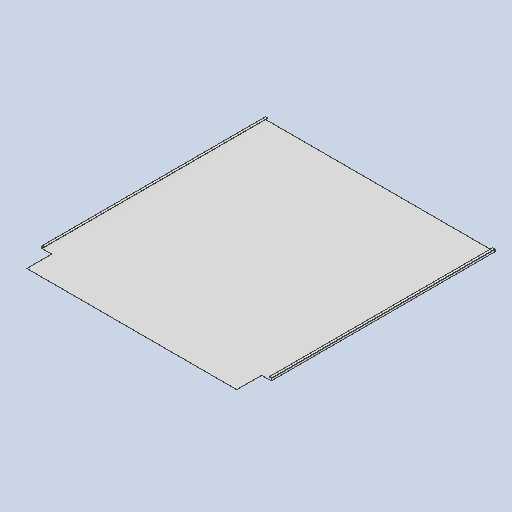
# Autodesk Inventor part: MSC 0201 sheet gills
Saved by Autodesk Inventor 2025 (Build 290162010, 162A)
## iProperties
Created: 2024-06-15
Part Number: MSC 0201 sheet gills
Material: Stainless Steel
Document SubType Name: Sheet Metal
Designer: pokla
Stock Number: МОО 0101 лист жабра
Mass: 7357.89 g
Surface Area: 36818.7 cm^2
Volume: 919.736 cm^3
Density: 8 g/cm^3
Flat Pattern Width: 96.1524 cm
Flat Pattern Length: 100 cm
Flat Pattern Area: 9615.24 cm^2
Sheet Metal Rule: Default_mm
Sheet Metal Width: 961,524 mm
Sheet Metal Length: 1000,000 mm
Sheet Metal Area: 961523,893 mm^2
Appearance: Default
Author: pokla
Autodesk Inventor part; units mm, degrees
ref_plane "YZ Plane" through (0, 0, 0) normal (1, 0, 0) x (0, 1, 0)
ref_plane "XZ Plane" through (0, 0, 0) normal (0, 1, 0) x (-1, 0, 0)
ref_plane "XY Plane" through (0, 0, 0) normal (0, 0, 1) x (1, 0, 0)
sketch "Sketch6" plane through (0, 0, 0) normal (0, 1, 0) x (-1, 0, 0)
  line L0 (462.5, -500) -> (-462.5, -500)
  line L1 (-462.5, -500) -> (-462.5, 500)
  line L2 (-462.5, 500) -> (462.5, 500)
  line L3 (462.5, 500) -> (462.5, -500)
  line L4 (462.5, -500) -> (-462.5, 500) construction
  line L5 (-462.5, -500) -> (462.5, 500) construction
  point P0 (0, 0)
  dimension "d52" = 925
  dimension "d53" = 1000
  measures "d52" distance of L1.end L2.end
  measures "d53" distance of L0.end L1.end
extrude "Plate2" add sketch "Sketch6" along normal blind 0.5
sketch "Sketch10" plane through (-462, 0, 500) normal (-1, 0, 0) x (0, -1, 0)
  line L0 (0, -1000) -> (0, 0)
  line L1 (0, 0) -> (-10, 0)
  line L2 (-10, 0) -> (-10, -1000)
  line L3 (-10, -1000) -> (0, -1000)
  constraints: 6 end point, 1 horizontal, 1 perpendicular, 1 vertical
edge flange "Flange1" height 10 angle 90 thickness 0.5 bend radius 0.5 thickness toward (-1, 0, 0) relief straight relief width 0.5 relief depth 0.25 corner gap 0.5 corner form 0 edges at (-462.5, 0.5, 0) (462.5, 0.5, 0) wall of the first edge with corners at (-462, 0, -500) (-462, 0, 500) (-462, 10, 500) (-462, 10, -500)
bend "Bend2"
corner "Corner2"
sketch "Sketch11" plane through (462.5, 9.5, -500) normal (0, 1, 0) x (-1, 0, 0)
  line L0 (0, 1000) -> (0, 0)
  line L1 (0, 0) -> (10, 0)
  line L2 (10, 0) -> (10, 1000)
  line L3 (10, 1000) -> (0, 1000)
  constraints: 6 end point, 1 horizontal, 1 perpendicular, 1 vertical
edge flange "Flange2" height 10 angle 90 thickness 0.5 bend radius 0.5 thickness toward (0, 1, 0) relief straight relief width 0.5 relief depth 0.25 corner gap 0.5 corner form 0 edges at (462, 10, 0) (-462, 10, 0) wall of the first edge with corners at (462.5, 9.5, 500) (462.5, 9.5, -500) (452.5, 9.5, -500) (452.5, 9.5, 500)
bend "Bend3"
corner "Corner3"
sketch "Sketch12" plane through (0, 0, 0) normal (0, -1, 0) x (1, 0, 0)
  line L0 (462.5, -500) -> (462.5, 500) projected
  line L1 (462.5, 500) -> (462.5, -500) projected
  line L2 (-462.5, -500) -> (-462.5, 500) projected
  line L3 (-462.5, 500) -> (-422.5, 500)
  line L4 (-422.5, 500) -> (-422.5, 400)
  line L5 (-422.5, 400) -> (-462.5, 400)
  line L6 (-462.5, 400) -> (-462.5, 500)
  line L7 (462.5, 500) -> (422.5, 500)
  line L8 (422.5, 500) -> (422.5, 400)
  line L9 (422.5, 400) -> (462.5, 400)
  line L10 (462.5, 400) -> (462.5, 500)
  point P0 (0, 0)
  point P1 (-462.5, 20.3845)
  dimension "d96" = 100
  dimension "d97" = 40
  dimension "d98" = 100
  dimension "d99" = 40
  constraints: 16 end point, 4 parallel, 2 horizontal, 2 perpendicular, 1 point on line
  measures "d96" distance between parallel lines of L3 L5
  measures "d97" distance of L4.end L5.end
  measures "d98" distance between parallel lines of L7 L9
  measures "d99" distance of L8.end L9.end
extrude "Extrusion3" cut sketch "Sketch12" along normal through all both and the other way through all
equation "\"d52\" = ЖАБРЫ_базовая_ширина"
equation "\"d53\" = ЖАБРЫ_базовая_длина_кор_лист"
equation "\"d98\" = d96"
equation "\"d99\" = d97"
equation "\"d54\" = Thickness"
equation "\"d74\" = BendReliefWidth"
equation "\"d75\" = BendReliefDepth"
equation "\"d76\" = MinimumRemnant"
equation "\"d77\" = TransitionRadius"
equation "\"d80\" = BendRadius"
equation "\"d81\" = CornerReliefSize"
equation "\"d82\" = GapSize"
equation "\"d83\" = JacobiRadiusSize"
equation "\"d84\" = BendReliefWidth"
equation "\"d85\" = BendReliefDepth"
equation "\"d86\" = MinimumRemnant"
equation "\"d87\" = TransitionRadius"
equation "\"d90\" = BendRadius"
equation "\"d91\" = CornerReliefSize"
equation "\"d92\" = GapSize"
equation "\"d93\" = JacobiRadiusSize"
equation "\"BendRadius\" = Thickness"
equation "\"BendReliefWidth\" = Thickness"
equation "\"BendReliefDepth\" = 0.5 * Thickness"
equation "\"CornerReliefSize\" = 4 * Thickness"
equation "\"MinimumRemnant\" = 2 * Thickness"
equation "\"TransitionRadius\" = BendRadius"
equation "\"JacobiRadiusSize\" = BendRadius"
equation "\"GapSize\" = Thickness"
equation "\"ЖАБРЫ_базовая_ширина\" = 925"
equation "\"ЖАБРЫ_базовая_длина_кор_лист\" = 1000"
equation "\"Thickness\" = 0.5"
body "Solid2"
